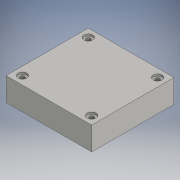
# Autodesk Inventor part: NUCBasePCB
Saved by Autodesk Inventor 2016 (Build 200138000, 138)
## iProperties
Created: 2015-09-23
Part Number: NUCBasePCB
Material: Generic
Document SubType Name: Modeling
Designer: lachesis
Density: 1 g/cm^3
Appearance: Default
Author: lachesis
Autodesk Inventor part; units mm, degrees
ref_plane "YZ Plane" through (0, 0, 0) normal (1, 0, 0) x (0, 1, 0)
ref_plane "XZ Plane" through (0, 0, 0) normal (0, 1, 0) x (-1, 0, 0)
ref_plane "XY Plane" through (0, 0, 0) normal (0, 0, 1) x (1, 0, 0)
sketch "Sketch1" plane through (0, 0, 0) normal (0, 1, 0) x (-1, 0, 0)
  line L0 (56.134, 58.42) -> (-56.134, 58.42)
  line L1 (-56.134, 58.42) -> (-56.134, -58.42)
  line L2 (-56.134, -58.42) -> (56.134, -58.42)
  line L3 (56.134, -58.42) -> (56.134, 58.42)
  point P0 (0, 0)
  point P1 (0, -58.42)
  point P2 (56.134, 0)
  dimension "d0" = 116.84
  dimension "d1" = 112.268
  constraints: 8 end point, 2 midpoint, 2 parallel, 1 horizontal, 1 horizontal alignment, 1 perpendicular, 1 vertical alignment
  measures "d0" distance of L2.end L0.start
  measures "d1" distance of L1.end L2.end
extrude "Extrusion1" add sketch "Sketch1" along normal blind 31.75
sketch "Sketch2" plane through (0, 31.75, 0) normal (0, 1, 0) x (1, 0, 0)
  line L0 (56.134, -58.42) -> (56.134, 58.42) projected
  line L1 (56.134, 58.42) -> (-56.134, 58.42) projected
  line L2 (-56.134, -58.42) -> (56.134, -58.42) projected
  line L3 (-56.134, 58.42) -> (-56.134, -58.42) projected
  point P0 (0, 0)
  point P1 (44.958, 47.244)
  point P2 (44.958, -47.244)
  point P3 (-44.958, 47.244)
  point P4 (-44.958, -47.244)
  dimension "d4" = 11.176
  dimension "d5" = 11.176
  dimension "d6" = 11.176
  dimension "d7" = 11.176
  constraints: 2 horizontal alignment, 2 vertical alignment
  measures "d4" distance from line of L0 point (44.958, 47.244)
  measures "d5" distance from line of L1 point (44.958, 47.244)
  measures "d6" distance from line of L2 point (-44.958, -47.244)
  measures "d7" distance from line of L3 point (-44.958, -47.244)
hole "Hole1" at (44.958, 31.75, -47.244) at (44.958, 31.75, 47.244) at (-44.958, 31.75, -47.244) at (-44.958, 31.75, 47.244) direction (0, -1, 0) diameter 3.302 end through all counterbore diameter 5.969 counterbore depth 26.162
sketch "Sketch3" plane through (0, 31.75, 0) normal (0, 1, 0) x (1, 0, 0)
  circle A0 centre (44.958, 47.244) radius 2.9845 projected
  circle A1 centre (44.958, -47.244) radius 2.9845 projected
  circle A2 centre (-44.958, 47.244) radius 2.9845 projected
  circle A3 centre (-44.958, -47.244) radius 2.9845 projected
  circle A4 centre (44.958, 47.244) radius 1.651 projected
  circle A5 centre (44.958, -47.244) radius 1.651 projected
  circle A6 centre (-44.958, -47.244) radius 1.651 projected
  point P0 (0, 0)
  constraints: 4 coincident
hole "Hole2" at (44.958, 31.75, -47.244) at (44.958, 31.75, 47.244) at (-44.958, 31.75, 47.244) at (-44.958, 31.75, -47.244) direction (0, -1, 0) diameter 12.065 depth 2.413
equation "\"d5\" = d4"
equation "\"d6\" = d4"
equation "\"d7\" = d4"
body "Solid1"
